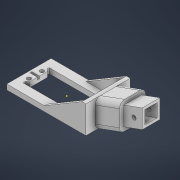
# Autodesk Inventor part: Servohalterung_v2
Saved by Autodesk Inventor 2021 (Build 250183000, 183)
## iProperties
Created: 2021-01-09
Part Number: Servohalterung_v2
Material: Generisch
Document SubType Name: Modeling
Designer: laure
Density: 1 g/cm^3
Appearance: Vorgabe
Author: laure
## iProperties of the stored document _3D-Druck.ipt
Created: 2021-01-22
Part Number: _3D-Druck
Material: Generisch
Document SubType Name: Modeling
Designer: Ctroi
Density: 1 g/cm^3
Appearance: Vorgabe
Author: Ctroi
Autodesk Inventor part; units mm, degrees
ref_plane "YZ Plane" through (0, 0, 0) normal (1, 0, 0) x (0, 1, 0)
ref_plane "XZ Plane" through (0, 0, 0) normal (0, 1, 0) x (-1, 0, 0)
ref_plane "XY Plane" through (0, 0, 0) normal (0, 0, 1) x (1, 0, 0)
sketch "Skizze1" plane through (0, 0, 0) normal (0, 1, 0) x (-1, 0, 0)
  line L0 (20.5, -10.1) -> (-20.5, -10.1)
  line L1 (-20.5, -10.1) -> (-20.5, 10.1)
  line L2 (-20.5, 10.1) -> (20.5, 10.1)
  line L3 (20.5, 10.1) -> (20.5, -10.1)
  line L4 (0, -23.94) -> (0, 23.94) projected
  line L5 (-40.6, 0) -> (40.6, 0) projected
  line L6 (29, -17.1) -> (-29, -17.1)
  line L7 (-29, -17.1) -> (-29, 17.1)
  line L8 (-29, 17.1) -> (29, 17.1)
  line L9 (29, 17.1) -> (29, -17.1)
  point P0 (0, 0)
  dimension "d0" = 41
  dimension "d3" = 20.2
  dimension "d7" = 58
  dimension "d8" = 7
  constraints: 16 end point, 4 parallel, 2 horizontal, 2 perpendicular, 4 other
  measures "d0" distance between parallel lines of L1 L3
  measures "d3" distance of L2.end L0.start
  measures "d7" distance between parallel lines of L7 L9
  measures "d8" distance between parallel lines of L6 L0
extrude "Extrusion2" add sketch "Skizze1" along normal mid plane 4 contours L3 L5 L9 L6 L4 L0 | L4 L6 L7 L5 L1 L0 | L3 L2 L4 L8 L9 L5 | L5 L7 L8 L4 L2 L1
sketch "Skizze2" plane through (0, 2, 0) normal (0, 1, 0) x (1, 0, 0)
  circle A0 centre (-24, 5) radius 1.55
  circle A1 centre (-24, -5) radius 1.55
  line L0 (-29, 17.1) -> (-29, -17.1) projected
  line L1 (40.6, 0) -> (-40.6, 0) projected
  line L2 (0, 23.94) -> (0, -23.94) projected
  circle A2 centre (24, 5) radius 1.55
  circle A3 centre (24, -5) radius 1.55
  line L3 (-20.5, -10.1) -> (-20.5, 10.1) projected
  point P0 (0, 0)
  dimension "d11" = 3.1
  dimension "d12" = 3.1
  dimension "d15" = 10
  dimension "d16" = 5
  dimension "d70" = 5
  dimension "d71" = 5
  constraints: 4 centre point, 2 symmetric about line, 2 other
  measures "d11" diameter of A0
  measures "d12" diameter of A1
  measures "d15" distance of A1.centre A0.centre
  measures "d16" distance from line of L1 A0.centre
  measures "d70" distance from line of L0 A0.centre
  measures "d71" distance from line of L0 A1.centre
extrude "Extrusion3" cut sketch "Skizze2" against normal up to surface (4 mm away)
sketch "Skizze3" plane through (0, 2, 0) normal (0, 1, 0) x (1, 0, 0)
  line L0 (-20.5, -10.1) -> (-20.5, 10.1) projected
  line L1 (-20.5, -0.75) -> (-27.5, -0.75)
  line L2 (-27.5, -0.75) -> (-27.5, 0.75)
  line L3 (-27.5, 0.75) -> (-20.5, 0.75)
  line L4 (-20.5, 0.75) -> (-20.5, -0.75)
  line L5 (40.6, 0) -> (-40.6, 0) projected
  line L6 (0, 23.94) -> (0, -23.94) projected
  line L7 (20.5, 10.1) -> (20.5, -10.1) projected
  line L8 (20.5, 0.75) -> (27.5, 0.75)
  line L9 (27.5, 0.75) -> (27.5, -0.75)
  line L10 (27.5, -0.75) -> (20.5, -0.75)
  line L11 (20.5, -0.75) -> (20.5, 0.75)
  point P0 (0, 0)
  dimension "d19" = 7
  dimension "d20" = 1.5
  dimension "d23" = 7
  constraints: 16 end point, 4 parallel, 2 horizontal, 2 perpendicular, 2 point on line, 2 other
  measures "d19" distance of L2.end L3.end
  measures "d20" distance of L1.end L2.end
  measures "d23" distance of L9.end L10.end
extrude "Extrusion4" cut sketch "Skizze3" against normal blind 2 contours L1 L2 L5 L0 | L5 L2 L3 L0
extrude "Extrusion5" cut sketch "Skizze3" against normal blind 2 contours L9 L10 L7 L5 | L5 L7 L8 L9
sketch "Skizze4" plane through (0, 0, 0) normal (0, 0, 1) x (1, 0, 0)
  line L0 (0, 33.8901) -> (0, -7.9817) projected
  line L1 (-13.0217, 0) -> (78.13, 0) projected
  line L2 (29, 2) -> (29, -2) projected
  line L3 (29, -2) -> (32, -2)
  line L4 (32, -2) -> (32, 19.216)
  line L5 (32, 19.216) -> (29, 19.216)
  line L6 (29, 19.216) -> (29, -2)
  line L7 (32, -2) -> (50.7939, 4.8404)
  line L8 (50.7939, 4.8404) -> (50.7939, 26.0564)
  line L9 (50.7939, 26.0564) -> (32, 19.216)
  line L10 (32, 15.858) -> (48.1939, 21.7521)
  line L11 (48.0492, 7.1994) -> (32, 1.358)
  line L12 (48.1939, 21.7521) -> (65.1083, 27.9084)
  line L13 (65.1083, 27.9084) -> (65.1083, 13.4084)
  line L14 (65.1083, 13.4084) -> (48.0492, 7.1994)
  line L15 (50.7939, 15.4484) -> (37.5768, 10.6378)
  line L16 (50.7939, 15.4484) -> (64.8591, 15.4484) construction
  point P0 (0, 0)
  point P1 (50.7939, 22.6984)
  point P2 (50.7939, 8.1984)
  dimension "d26" = 3
  dimension "d27" = 21.216
  dimension "d28" = 20
  dimension "d29" = 21.216
  dimension "d30" = 20
  dimension "d38" = 110
  dimension "d42" = 18
  dimension "d44" = 110
  dimension "d48" = 14.3145
  dimension "d66" = 14.5
  dimension "d67" = 160
  constraints: 28 end point, 3 parallel, 2 horizontal, 2 point on line, 2 vertical, 1 equal length, 1 midpoint, 1 perpendicular, 1 other
  measures "d26" distance of L5.end L4.end
  measures "d27" distance of L4.end L3.end
  measures "d28" distance of L3.end L7.end
  measures "d29" distance of L7.end L8.end
  measures "d30" angle of L9 L5
  measures "d38" angle of L11 L4
  measures "d42" distance of L10.end L12.end
  measures "d44" angle of L13 L14
  measures "d48" distance between parallel lines of L8 L13
  measures "d66" distance of L11.end L10.start
  measures "d67" angle of L15 L16
extrude "Extrusion6" add sketch "Skizze4" along normal mid plane 34.2 contours L2 L6 L5 L4 L1 | L1 L4 L3 L2
sketch "Skizze6" plane through (0, 0, 0) normal (0, 0, 1) x (1, 0, 0)
  point P0 (0, 0)
extrude "Extrusion7" add sketch "Skizze4" along normal mid plane 20 contours L4 L11 L14 L8 L7 L1 | L1 L7 L4 | L4 L10 L12 L8 L14 L11 | L4 L9 L8 L12 L10
extrude "Extrusion9" add sketch "Skizze4" along normal mid plane 13.5 contours L8 L12 L13 L14
shell "Wandung2" thickness 2 removed faces 1 at (65.1083, 18.2418, -2.25)
fillet "Rundung1" radius 4 4 edges at (41.3969, 22.6362, 10) (41.3969, 22.6362, -10) (41.3969, 1.4202, -10) (41.3969, 1.4202, 10)
sketch "Skizze7" plane through (-29, -2, 17.1) normal (0, 0, 1) x (1, 0, 0)
  line L0 (-12.2, 2) -> (73.2, 2) projected
  line L1 (29, 25.4592) -> (29, -4.2432) projected
  line L2 (58, 4) -> (58, 21.216) projected
  line L3 (58, 21.216) -> (29, 4)
  line L4 (8.5, 4) -> (49.5, 4) projected
  line L5 (58, 4) -> (0, 4) projected
  line L6 (58, 4) -> (58, 21.216)
  point P0 (29, 2)
  constraints: 4 end point, 1 midpoint, 1 vertical
extrude "Extrusion10" add sketch "Skizze7" against normal blind 2
sketch "Skizze8" plane through (-29, -2, -17.1) normal (0, 0, -1) x (-1, 0, 0)
  line L0 (-29, -4.2432) -> (-29, 25.4592) projected
  line L1 (-73.2, 2) -> (12.2, 2) projected
  line L2 (-58, 4) -> (-58, 21.216) projected
  line L3 (-58, 21.216) -> (-29, 4)
  line L4 (-8.5, 4) -> (-49.5, 4) projected
  line L5 (-58, 4) -> (0, 4) projected
  line L6 (-58, 21.216) -> (-61, 21.216) projected
  line L7 (-58, 4) -> (-58, 21.216)
  point P0 (-29, 2)
  constraints: 4 end point, 1 midpoint, 1 vertical
extrude "Extrusion11" add sketch "Skizze8" against normal blind 2
sketch "Skizze9" plane through (0, 0, 6.75) normal (0, 0, 1) x (1, 0, 0)
  circle A0 centre (58.7939, 18.3602) radius 1.6
  line L0 (65.1083, 13.4084) -> (65.1083, 27.9084) projected
  line L1 (65.1083, 15.5368) -> (65.1083, 25.7801) projected
  line L2 (65.1083, 20.6584) -> (53.7155, 16.5118)
  line L3 (65.1083, 20.6584) -> (77.2323, 20.6584) construction
  line L4 (50.7939, 8.1984) -> (50.7939, 22.6984) projected
  point P0 (0, 0)
  dimension "d60" = 3.2
  dimension "d62" = 160
  dimension "d63" = 8
  constraints: 4 end point, 1 centre point, 1 equal length, 1 horizontal, 1 midpoint, 1 point on line
  measures "d60" diameter of A0
  measures "d62" angle of L2 L3
  measures "d63" distance from line of L4 A0.centre
extrude "Extrusion12" cut sketch "Skizze9" against normal up to surface (13.5 mm away)
sketch "Skizze11" plane through (0, 2, 0) normal (0, 1, 0) x (1, 0, 0)
  line L0 (-20.5, 10.1) -> (-23.5, 10.1)
  line L1 (-23.5, 10.1) -> (-23.5, 8.325)
  line L2 (-20.5, 0) -> (-20.5, 10.1)
  line L3 (-23.5, 8.325) -> (-21.7, 7.02)
  line L4 (0, 23.94) -> (0, -23.94) projected
  line L5 (83.93, 0) -> (-47.8217, 0) projected
  line L6 (-21.7, 7.02) -> (-21.7, 0)
  line L7 (-20.5, 0.75) -> (-20.5, -0.75) projected
  line L8 (-20.5, 0) -> (-20.5, 10.1)
  line L9 (-20.5, 0.75) -> (-20.5, 10.1) projected
  line L10 (-21.7, 0) -> (-20.5, 0)
  line L11 (-20.5, -10.1) -> (-23.5, -10.1)
  line L12 (-23.5, -10.1) -> (-23.5, -8.325)
  line L13 (-20.5, 0) -> (-20.5, -10.1)
  line L14 (-23.5, -8.325) -> (-21.7, -7.02)
  line L15 (-21.7, -7.02) -> (-21.7, 0)
  line L16 (-20.5, 0) -> (-20.5, -10.1)
  line L17 (-20.5, -0.75) -> (-20.5, -10.1)
  line L18 (20.5, 10.1) -> (23.5, 10.1)
  line L19 (23.5, 10.1) -> (23.5, 8.325)
  line L20 (20.5, 0) -> (20.5, 10.1)
  line L21 (23.5, 8.325) -> (21.7, 7.02)
  line L22 (21.7, 7.02) -> (21.7, 0)
  line L23 (20.5, 0.75) -> (20.5, -0.75)
  line L24 (20.5, 0) -> (20.5, 10.1)
  line L25 (20.5, 0.75) -> (20.5, 10.1)
  line L26 (21.7, 0) -> (20.5, 0)
  line L27 (20.5, -10.1) -> (23.5, -10.1)
  line L28 (23.5, -10.1) -> (23.5, -8.325)
  line L29 (20.5, 0) -> (20.5, -10.1)
  line L30 (23.5, -8.325) -> (21.7, -7.02)
  line L31 (21.7, -7.02) -> (21.7, 0)
  line L32 (20.5, 0) -> (20.5, -10.1)
  line L33 (20.5, -0.75) -> (20.5, -10.1)
  point P0 (0, 0)
  dimension "d81" = 3
  dimension "d82" = 1.2
  dimension "d83" = 54.058
  dimension "d84" = 14.1075
  constraints: 60 end point, 19 symmetric about line, 5 point on line, 2 collinear, 2 perpendicular, 1 horizontal, 1 midpoint, 1 parallel
  measures "d81" distance between parallel lines of L2 L1
  measures "d82" distance between parallel lines of L2 L6
  measures "d83" angle of L4 L14
  measures "d84" distance between parallel lines of L21 L14
extrude "Extrusion14" cut sketch "Skizze11" against normal up to surface (4 mm away)
sketch "Skizze12" plane through (0, 0, 0) normal (0, 0, 1) x (1, 0, 0)
  line L0 (23.5, 2) -> (-23.5, 2) projected
  line L1 (-7.3323, 2) -> (70.674, 2)
  line L2 (70.674, 2) -> (70.674, 29.3294)
  line L3 (70.674, 29.3294) -> (-7.3323, 29.3294)
  line L4 (-7.3323, 29.3294) -> (-7.3323, 2)
  line L5 (32, -2) -> (50.7939, 4.8404) projected
  line L6 (32, -2) -> (54.6251, -2)
  line L7 (54.6251, -2) -> (54.6251, 2)
  line L8 (54.6251, 2) -> (32, 2)
  line L9 (32, 2) -> (32, -2)
  point P0 (0, 0)
  constraints: 16 end point, 4 parallel, 2 horizontal, 2 perpendicular, 2 point on line
sketch "Skizze10" plane through (0, 0, 0) normal (0, 0, 1) x (1, 0, 0)
  line L0 (-46.9108, 47.129) -> (37.4559, 47.129)
  line L1 (37.4559, 47.129) -> (37.4559, -27.201)
  line L2 (37.4559, -27.201) -> (-46.9108, -27.201)
  line L3 (-46.9108, -27.201) -> (-46.9108, 47.129)
  point P0 (0, 0)
  constraints: 8 end point, 2 parallel, 1 horizontal, 1 perpendicular
